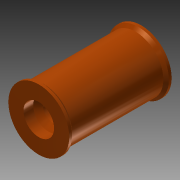
# Autodesk Inventor part: spool holder
Saved by Autodesk Inventor 2013 (Build 170138000, 138)
## iProperties
Created: 2013-07-29
Part Number: spool holder
Material: Generic
Document SubType Name: Modeling
Designer: employee
Density: 1 g/cm^3
Mass: 37.0145 g
Surface Area: 192.303 cm^2
Volume: 37.0145 cm^3
Author: employee
Autodesk Inventor part; units mm, degrees
ref_plane "YZ Plane" through (0, 0, 0) normal (1, 0, 0) x (0, 1, 0)
ref_plane "XZ Plane" through (0, 0, 0) normal (0, 1, 0) x (-1, 0, 0)
ref_plane "XY Plane" through (0, 0, 0) normal (0, 0, 1) x (1, 0, 0)
sketch "Sketch1" plane through (0, 0, 0) normal (1, 0, 0) x (0, 1, 0)
  line L0 (0, 0) -> (0, 22)
  line L1 (0, 22) -> (2, 22)
  line L2 (2, 22) -> (2, 20)
  line L3 (2, 20) -> (72, 20)
  line L4 (72, 20) -> (72, 22)
  line L5 (72, 22) -> (74, 22)
  line L6 (74, 22) -> (74, 0)
  line L7 (74, 0) -> (0, 0)
  point P0 (74, 11)
  dimension "d0" = 22
  dimension "d5" = 70
  dimension "d6" = 2
  dimension "d7" = 2
  dimension "d29" = 2
  constraints: 16 end point, 3 parallel, 1 collinear, 1 horizontal, 1 midpoint, 1 perpendicular, 1 point on line, 1 vertical, 1 vertical alignment
  measures "d0" distance between parallel lines of L7 L5
  measures "d5" distance of L2.end L3.end
  measures "d6" distance of L0.end L1.end
  measures "d7" distance of L4.end L5.end
  measures "d29" distance between parallel lines of L1 L3
revolve "Revolution1" add sketch "Sketch1" angle 360 about axis through (0, 74, 0) along (0, -1, 0)
chamfer "Chamfer1" distance 2 angle 45 2 edges at (0, 2, -20) (0, 72, -20)
sketch "Sketch2" plane through (0, 74, 0) normal (0, 1, 0) x (1, 0, 0)
  circle A0 centre (0, 0) radius 22 projected
  circle A1 centre (0, 0) radius 11.05
  dimension "d12" = 22.1
  constraints: 1 centre point, 1 coincident
  measures "d12" diameter of A1
extrude "Extrusion1" cut sketch "Sketch2" against normal blind 56 contours A1
sketch "Sketch3" plane through (0, 0, 0) normal (0, -1, 0) x (1, 0, 0)
  circle A0 centre (0, 0) radius 22 projected
  circle A1 centre (0, 0) radius 11.05 projected
extrude "Extrusion2" cut sketch "Sketch3" against normal blind 7 contours A1
sketch "Sketch4" plane through (0, 7, 0) normal (0, -1, 0) x (1, 0, 0)
  circle A0 centre (0, 0) radius 11.05 projected
  circle A1 centre (0, 0) radius 7.55
  dimension "d18" = 15.1
  constraints: 1 centre point, 1 coincident
  measures "d18" diameter of A1
extrude "Extrusion3" cut sketch "Sketch4" against normal through all contours A1
chamfer "Chamfer2" distance 3.5 angle 45 1 edges at (-7.55, 7, 0)
sketch "Sketch5" plane through (0, 74, 0) normal (0, 1, 0) x (1, 0, 0)
  circle A0 centre (0, 0) radius 11.05 projected
  circle A1 centre (0, 0) radius 20 projected
  circle A2 centre (0, 0) radius 18
  dimension "d25" = 8.95
  dimension "d26" = 2
  constraints: 1 centre point, 1 coincident
  measures "d25" radial gap between concentric circles of A1 A0
  measures "d26" radial gap between concentric circles of A1 A2
extrude "Extrusion4" cut sketch "Sketch5" against normal blind 49 contours A2
body "Solid1"
